Faucet Spacer (Autodesk Fusion 360 design; units mm, degrees)
Autodesk Fusion 360 part; units mm, degrees
sketch "Sketch1" plane through (0, 0, 0) normal (0, 0, 1) x (1, 0, 0)
  circle A0 centre (0, 0) radius 18
  circle A1 centre (0, 0) radius 13.5
  dimension "d1" = 36
  dimension "d2" = 4.5
  constraint coincident A0.centre A1.centre
  constraint concentric A0 A1
  measures "d1" diameter of A0
  measures "d2" distance of A0 A1
extrude "Extrude1" add sketch "Sketch1" along normal blind 4
ref_plane "WorkPlane1" through (0, 0, 2) normal (0, 0, 1) x (1, 0, 0)
sketch "Sketch2" plane through (0, 0, 0) normal (0, 1, 0) x (1, 0, 0)
  line L0 (-18, -4) -> (18, -2)
  line L1 (-18, 0) -> (18, 0)
  line L2 (18, -2) -> (19.6734, -6.6773)
  line L3 (19.6734, -6.6773) -> (-20, -6.6773)
  line L4 (-20, -6.6773) -> (-18, -4)
  dimension "d6" = 2
  dimension "d7" = 4
  constraint horizontal L3
  measures "d6" distance of L0.end L1
  measures "d7" distance of L0.start L1
extrude "Extrude2" cut sketch "Sketch2" along normal mid plane 42
